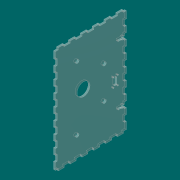
# Autodesk Inventor part: leftSide
Saved by Autodesk Inventor 2016 (Build 200138000, 138)
## iProperties
Created: 2015-10-05
Part Number: leftSide
Material: Polycarbonate, Clear
Document SubType Name: Modeling
Designer: Sawaiz
Density: 1.2 g/cm^3
Appearance: Polycarbonate - Clear
Author: Sawaiz
Autodesk Inventor part; units mm, degrees
ref_plane "YZ Plane" through (0, 0, 0) normal (1, 0, 0) x (0, 1, 0)
ref_plane "XZ Plane" through (0, 0, 0) normal (0, 1, 0) x (-1, 0, 0)
ref_plane "XY Plane" through (0, 0, 0) normal (0, 0, 1) x (1, 0, 0)
sketch "Sketch1" plane through (0, 0, 0) normal (1, 0, 0) x (0, 1, 0)
  line L0 (-56.825, -86.825) -> (56.825, -86.825)
  line L1 (56.825, -86.825) -> (56.825, 86.825)
  line L2 (56.825, 86.825) -> (-56.825, 86.825)
  line L3 (-56.825, 86.825) -> (-56.825, -86.825)
  line L4 (-56.825, -86.825) -> (56.825, 86.825) construction
  line L5 (56.825, -86.825) -> (-56.825, 86.825) construction
  point P0 (0, 0)
  dimension "d0" = 113.65
  dimension "d1" = 173.65
  constraints: 12 end point, 2 midpoint, 2 parallel, 1 horizontal, 1 perpendicular
  measures "d0" distance of L2.end L1.end
  measures "d1" distance of L1.end L0.end
extrude "Extrusion1" add sketch "Sketch1" along normal blind 3.175
sketch "Sketch10" plane through (0, 0, 0) normal (-1, 0, 0) x (0, 0, 1)
  line L0 (-86.825, -56.825) -> (-86.825, 56.825) projected
  line L1 (86.825, -56.825) -> (-86.825, -56.825) projected
  line L2 (86.825, 56.825) -> (86.825, -56.825) projected
  line L3 (-86.825, 56.825) -> (86.825, 56.825) projected
  line L4 (86.825, 56.825) -> (86.825, -56.825) projected
  line L5 (86.825, -55) -> (90, -55)
  line L6 (90, -55) -> (90, -45)
  line L7 (90, -45) -> (86.825, -45)
  line L8 (86.825, -45) -> (86.825, -55)
  point P0 (0, 0)
  dimension "d84" = 10
  dimension "d85" = 1.825
  dimension "d86" = 3.175
  constraints: 8 end point, 2 parallel, 1 horizontal, 1 perpendicular, 1 point on line
  measures "d84" distance of L5.end L6.end
  measures "d85" distance between parallel lines of L1 L5
  measures "d86" distance of L6.end L7.end
extrude "Extrusion4" add sketch "Sketch10" against normal up to surface (3.175 mm away) contours L2 L7 L6 L5
pattern_linear "Rectangular Pattern3" count 6 spacing 20 along (0, 1, 0) of "Extrusion4"
mirror "Mirror3" about plane through (0, 0, 0) normal (0, 0, 1) of "Extrusion4", "Rectangular Pattern3"
sketch "Sketch11" plane through (0, 0, 0) normal (-1, 0, 0) x (0, 0, 1)
  line L0 (-86.825, -56.825) -> (-86.825, -55) projected
  line L1 (86.825, -56.825) -> (-86.825, -56.825) projected
  line L2 (86.825, -55) -> (86.825, -56.825) projected
  line L3 (86.825, -55) -> (90, -55) projected
  line L4 (90, -55) -> (90, -45) projected
  line L5 (90, -45) -> (86.825, -45) projected
  line L6 (86.825, -35) -> (86.825, -45) projected
  line L7 (86.825, -35) -> (90, -35) projected
  line L8 (90, -35) -> (90, -25) projected
  line L9 (90, -25) -> (86.825, -25) projected
  line L10 (86.825, -15) -> (86.825, -25) projected
  line L11 (86.825, -15) -> (90, -15) projected
  line L12 (90, -15) -> (90, -5) projected
  line L13 (90, -5) -> (86.825, -5) projected
  line L14 (86.825, 5) -> (86.825, -5) projected
  line L15 (86.825, 5) -> (90, 5) projected
  line L16 (90, 5) -> (90, 15) projected
  line L17 (90, 15) -> (86.825, 15) projected
  line L18 (86.825, 25) -> (86.825, 15) projected
  line L19 (86.825, 25) -> (90, 25) projected
  line L20 (90, 25) -> (90, 35) projected
  line L21 (90, 35) -> (86.825, 35) projected
  line L22 (86.825, 45) -> (86.825, 35) projected
  line L23 (86.825, 45) -> (90, 45) projected
  line L24 (90, 45) -> (90, 55) projected
  line L25 (90, 55) -> (86.825, 55) projected
  line L26 (-86.825, 56.825) -> (86.825, 56.825) projected
  line L27 (-90, 55) -> (-86.825, 55) projected
  line L28 (-90, 45) -> (-90, 55) projected
  line L29 (-86.825, 45) -> (-90, 45) projected
  line L30 (-86.825, 35) -> (-86.825, 45) projected
  line L31 (-90, 35) -> (-86.825, 35) projected
  line L32 (-90, 25) -> (-90, 35) projected
  line L33 (-86.825, 25) -> (-90, 25) projected
  line L34 (-86.825, 15) -> (-86.825, 25) projected
  line L35 (-90, 15) -> (-86.825, 15) projected
  line L36 (-90, 5) -> (-90, 15) projected
  line L37 (-86.825, 5) -> (-90, 5) projected
  line L38 (-86.825, -5) -> (-86.825, 5) projected
  line L39 (-90, -5) -> (-86.825, -5) projected
  line L40 (-90, -15) -> (-90, -5) projected
  line L41 (-86.825, -15) -> (-90, -15) projected
  line L42 (-86.825, -25) -> (-86.825, -15) projected
  line L43 (-90, -25) -> (-86.825, -25) projected
  line L44 (-90, -35) -> (-90, -25) projected
  line L45 (-86.825, -35) -> (-90, -35) projected
  line L46 (-86.825, -45) -> (-86.825, -35) projected
  line L47 (-90, -45) -> (-86.825, -45) projected
  line L48 (-90, -55) -> (-90, -45) projected
  line L49 (-86.825, -55) -> (-90, -55) projected
  line L50 (86.825, -56.825) -> (-86.825, -56.825) projected
  line L51 (85, -56.825) -> (75, -56.825)
  line L52 (75, -56.825) -> (75, -60)
  line L53 (75, -60) -> (85, -60)
  line L54 (85, -60) -> (85, -56.825)
  line L55 (86.825, 56.825) -> (86.825, 55) projected
  line L56 (-86.825, 55) -> (-86.825, 56.825) projected
  point P0 (0, 0)
  dimension "d92" = 3.175
  dimension "d94" = 10
  dimension "d100" = 5
  constraints: 8 end point, 2 parallel, 1 horizontal, 1 perpendicular, 1 point on line
  measures "d92" distance of L53.end L51.start
  measures "d94" distance of L52.end L53.end
  measures "d100" distance between parallel lines of L4 L54
extrude "Extrusion5" add sketch "Sketch11" against normal up to surface (3.175 mm away) contours L1 L54 L53 L52
pattern_linear "Rectangular Pattern4" count 9 spacing 20 along (0, 0, -1) of "Extrusion5"
sketch "Sketch16" plane through (3.175, 0, 0) normal (1, 0, 0) x (0, 0, -1)
  line L0 (86.825, -56.825) -> (86.825, -55) projected
  line L1 (86.825, -55) -> (90, -55) projected
  line L2 (90, -55) -> (90, -45) projected
  line L3 (90, -45) -> (86.825, -45) projected
  line L4 (86.825, -45) -> (86.825, -35) projected
  line L5 (86.825, -35) -> (90, -35) projected
  line L6 (90, -35) -> (90, -25) projected
  line L7 (90, -25) -> (86.825, -25) projected
  line L8 (86.825, -25) -> (86.825, -15) projected
  line L9 (86.825, -15) -> (90, -15) projected
  line L10 (90, -15) -> (90, -5) projected
  line L11 (90, -5) -> (86.825, -5) projected
  line L12 (86.825, -5) -> (86.825, 5) projected
  line L13 (86.825, 5) -> (90, 5) projected
  line L14 (90, 5) -> (90, 15) projected
  line L15 (90, 15) -> (86.825, 15) projected
  line L16 (86.825, 15) -> (86.825, 25) projected
  line L17 (86.825, 25) -> (90, 25) projected
  line L18 (90, 25) -> (90, 35) projected
  line L19 (90, 35) -> (86.825, 35) projected
  line L20 (86.825, 35) -> (86.825, 45) projected
  line L21 (86.825, 45) -> (90, 45) projected
  line L22 (90, 45) -> (90, 55) projected
  line L23 (90, 55) -> (86.825, 55) projected
  line L24 (86.825, 55) -> (86.825, 56.825) projected
  line L25 (86.825, 56.825) -> (-86.825, 56.825) projected
  line L26 (-86.825, 56.825) -> (-86.825, 55) projected
  line L27 (-90, 55) -> (-86.825, 55) projected
  line L28 (-90, 45) -> (-90, 55) projected
  line L29 (-86.825, 45) -> (-90, 45) projected
  line L30 (-86.825, 45) -> (-86.825, 35) projected
  line L31 (-90, 35) -> (-86.825, 35) projected
  line L32 (-90, 25) -> (-90, 35) projected
  line L33 (-86.825, 25) -> (-90, 25) projected
  line L34 (-86.825, 25) -> (-86.825, 15) projected
  line L35 (-90, 15) -> (-86.825, 15) projected
  line L36 (-90, 5) -> (-90, 15) projected
  line L37 (-86.825, 5) -> (-90, 5) projected
  line L38 (-86.825, 5) -> (-86.825, -5) projected
  line L39 (-90, -5) -> (-86.825, -5) projected
  line L40 (-90, -15) -> (-90, -5) projected
  line L41 (-86.825, -15) -> (-90, -15) projected
  line L42 (-86.825, -15) -> (-86.825, -25) projected
  line L43 (-90, -25) -> (-86.825, -25) projected
  line L44 (-90, -35) -> (-90, -25) projected
  line L45 (-86.825, -35) -> (-90, -35) projected
  line L46 (-86.825, -35) -> (-86.825, -45) projected
  line L47 (-90, -45) -> (-86.825, -45) projected
  line L48 (-90, -55) -> (-90, -45) projected
  line L49 (-86.825, -55) -> (-90, -55) projected
  line L50 (-86.825, -55) -> (-86.825, -56.825) projected
  line L51 (-86.825, -56.825) -> (-85, -56.825) projected
  line L52 (-85, -60) -> (-85, -56.825) projected
  line L53 (-75, -60) -> (-85, -60) projected
  line L54 (-75, -56.825) -> (-75, -60) projected
  line L55 (-75, -56.825) -> (-65, -56.825) projected
  line L56 (-65, -60) -> (-65, -56.825) projected
  line L57 (-55, -60) -> (-65, -60) projected
  line L58 (-55, -56.825) -> (-55, -60) projected
  line L59 (-55, -56.825) -> (-45, -56.825) projected
  line L60 (-45, -60) -> (-45, -56.825) projected
  line L61 (-35, -60) -> (-45, -60) projected
  line L62 (-35, -56.825) -> (-35, -60) projected
  line L63 (-35, -56.825) -> (-25, -56.825) projected
  line L64 (-25, -60) -> (-25, -56.825) projected
  line L65 (-15, -60) -> (-25, -60) projected
  line L66 (-15, -56.825) -> (-15, -60) projected
  line L67 (-15, -56.825) -> (-5, -56.825) projected
  line L68 (-5, -60) -> (-5, -56.825) projected
  line L69 (5, -60) -> (-5, -60) projected
  line L70 (5, -56.825) -> (5, -60) projected
  line L71 (5, -56.825) -> (15, -56.825) projected
  line L72 (15, -60) -> (15, -56.825) projected
  line L73 (25, -60) -> (15, -60) projected
  line L74 (25, -56.825) -> (25, -60) projected
  line L75 (25, -56.825) -> (35, -56.825) projected
  line L76 (35, -60) -> (35, -56.825) projected
  line L77 (45, -60) -> (35, -60) projected
  line L78 (45, -56.825) -> (45, -60) projected
  line L79 (45, -56.825) -> (55, -56.825) projected
  line L80 (55, -60) -> (55, -56.825) projected
  line L81 (65, -60) -> (55, -60) projected
  line L82 (65, -56.825) -> (65, -60) projected
  line L83 (65, -56.825) -> (75, -56.825) projected
  line L84 (75, -60) -> (75, -56.825) projected
  line L85 (85, -60) -> (75, -60) projected
  line L86 (85, -56.825) -> (85, -60) projected
  line L87 (85, -56.825) -> (86.825, -56.825) projected
  line L88 (-85, -56.825) -> (-86.825, -56.825)
  line L89 (-86.825, -56.825) -> (-86.825, -60)
  line L90 (-86.825, -60) -> (-85, -60)
  line L91 (-85, -60) -> (-85, -56.825)
  line L92 (85, -56.825) -> (85, -60) projected
  line L93 (85, -56.825) -> (86.825, -56.825)
  line L94 (86.825, -56.825) -> (86.825, -60)
  line L95 (86.825, -60) -> (85, -60)
  line L96 (85, -60) -> (85, -56.825)
  point P0 (0, 0)
  constraints: 16 end point, 4 collinear, 4 parallel, 2 horizontal, 2 perpendicular
extrude "Extrusion8" add sketch "Sketch16" against normal up to surface (3.175 mm away) contours L94 L95 L86 L87 | L90 L89 L51 L52
mirror "Mirror4" about plane through (0, 0, 0) normal (0, 1, 0) of "Extrusion5", "Rectangular Pattern4", "Extrusion8"
sketch "Sketch2" plane through (3.175, 0, 0) normal (1, 0, 0) x (0, 0, -1)
  line L0 (86.825, -60) -> (86.825, -55) projected
  line L1 (-65, 56.825) -> (-75, 56.825) projected
  line L2 (-86.825, 55) -> (-86.825, 60) projected
  line L3 (-75, -56.825) -> (-65, -56.825) projected
  line L4 (-86.825, 56.825) -> (-86.825, -56.825) projected
  line L5 (86.825, -55) -> (90, -55) projected
  line L6 (90, -55) -> (90, -45) projected
  line L7 (90, -45) -> (86.825, -45) projected
  line L8 (86.825, -45) -> (86.825, -35) projected
  line L9 (86.825, -35) -> (90, -35) projected
  line L10 (90, -35) -> (90, -25) projected
  line L11 (90, -25) -> (86.825, -25) projected
  line L12 (86.825, -15) -> (90, -15) projected
  line L13 (90, -15) -> (90, -5) projected
  line L14 (90, -5) -> (86.825, -5) projected
  line L15 (86.825, -5) -> (86.825, 5) projected
  line L16 (86.825, 5) -> (90, 5) projected
  line L17 (90, 5) -> (90, 15) projected
  line L18 (90, 15) -> (86.825, 15) projected
  line L19 (86.825, 15) -> (86.825, 25) projected
  line L20 (86.825, 25) -> (90, 25) projected
  line L21 (90, 25) -> (90, 35) projected
  line L22 (90, 35) -> (86.825, 35) projected
  line L23 (86.825, 35) -> (86.825, 45) projected
  line L24 (86.825, 45) -> (90, 45) projected
  line L25 (90, 45) -> (90, 55) projected
  line L26 (90, 55) -> (86.825, 55) projected
  line L27 (86.825, 60) -> (75, 60) projected
  line L28 (75, 60) -> (75, 56.825) projected
  line L29 (65, 56.825) -> (65, 60) projected
  line L30 (65, 60) -> (55, 60) projected
  line L31 (55, 60) -> (55, 56.825) projected
  line L32 (55, 56.825) -> (45, 56.825) projected
  line L33 (45, 56.825) -> (45, 60) projected
  line L34 (45, 60) -> (35, 60) projected
  line L35 (35, 60) -> (35, 56.825) projected
  line L36 (35, 56.825) -> (25, 56.825) projected
  line L37 (25, 56.825) -> (25, 60) projected
  line L38 (25, 60) -> (15, 60) projected
  line L39 (15, 60) -> (15, 56.825) projected
  line L40 (15, 56.825) -> (5, 56.825) projected
  line L41 (5, 56.825) -> (5, 60) projected
  line L42 (5, 60) -> (-5, 60) projected
  line L43 (-5, 60) -> (-5, 56.825) projected
  line L44 (-5, 56.825) -> (-15, 56.825) projected
  line L45 (-15, 56.825) -> (-15, 60) projected
  line L46 (-15, 60) -> (-25, 60) projected
  line L47 (-25, 60) -> (-25, 56.825) projected
  line L48 (-25, 56.825) -> (-35, 56.825) projected
  line L49 (-35, 56.825) -> (-35, 60) projected
  line L50 (-35, 60) -> (-45, 60) projected
  line L51 (-45, 60) -> (-45, 56.825) projected
  line L52 (-45, 56.825) -> (-55, 56.825) projected
  line L53 (-55, 56.825) -> (-55, 60) projected
  line L54 (-55, 60) -> (-65, 60) projected
  line L55 (-65, 60) -> (-65, 56.825) projected
  line L56 (-75, 56.825) -> (-75, 60) projected
  line L57 (-75, 60) -> (-86.825, 60) projected
  line L58 (-90, 55) -> (-86.825, 55) projected
  line L59 (-90, 45) -> (-90, 55) projected
  line L60 (-86.825, 45) -> (-90, 45) projected
  line L61 (-86.825, 45) -> (-86.825, 35) projected
  line L62 (-90, 35) -> (-86.825, 35) projected
  line L63 (-90, 25) -> (-90, 35) projected
  line L64 (-86.825, 25) -> (-90, 25) projected
  line L65 (-86.825, 25) -> (-86.825, 15) projected
  line L66 (-90, 15) -> (-86.825, 15) projected
  line L67 (-90, 5) -> (-90, 15) projected
  line L68 (-86.825, 5) -> (-90, 5) projected
  line L69 (-86.825, 5) -> (-86.825, -5) projected
  line L70 (-90, -5) -> (-86.825, -5) projected
  line L71 (-90, -15) -> (-90, -5) projected
  line L72 (-86.825, -15) -> (-90, -15) projected
  line L73 (-86.825, -15) -> (-86.825, -25) projected
  line L74 (-90, -25) -> (-86.825, -25) projected
  line L75 (-90, -35) -> (-90, -25) projected
  line L76 (-86.825, -35) -> (-90, -35) projected
  line L77 (-86.825, -35) -> (-86.825, -45) projected
  line L78 (-90, -45) -> (-86.825, -45) projected
  line L79 (-90, -55) -> (-90, -45) projected
  line L80 (-86.825, -55) -> (-90, -55) projected
  line L81 (-75, -60) -> (-86.825, -60) projected
  line L82 (-75, -56.825) -> (-75, -60) projected
  line L83 (-65, -60) -> (-65, -56.825) projected
  line L84 (-55, -60) -> (-65, -60) projected
  line L85 (-55, -56.825) -> (-55, -60) projected
  line L86 (-55, -56.825) -> (-45, -56.825) projected
  line L87 (-45, -60) -> (-45, -56.825) projected
  line L88 (-35, -60) -> (-45, -60) projected
  line L89 (-35, -56.825) -> (-35, -60) projected
  line L90 (-35, -56.825) -> (-25, -56.825) projected
  line L91 (-25, -60) -> (-25, -56.825) projected
  line L92 (-15, -60) -> (-25, -60) projected
  line L93 (-15, -56.825) -> (-15, -60) projected
  line L94 (-15, -56.825) -> (-5, -56.825) projected
  line L95 (-5, -60) -> (-5, -56.825) projected
  line L96 (5, -60) -> (-5, -60) projected
  line L97 (5, -56.825) -> (5, -60) projected
  line L98 (5, -56.825) -> (15, -56.825) projected
  line L99 (15, -60) -> (15, -56.825) projected
  line L100 (25, -60) -> (15, -60) projected
  line L101 (25, -56.825) -> (25, -60) projected
  line L102 (25, -56.825) -> (35, -56.825) projected
  line L103 (35, -60) -> (35, -56.825) projected
  line L104 (45, -60) -> (35, -60) projected
  line L105 (45, -56.825) -> (45, -60) projected
  line L106 (45, -56.825) -> (55, -56.825) projected
  line L107 (55, -60) -> (55, -56.825) projected
  line L108 (65, -60) -> (55, -60) projected
  line L109 (65, -56.825) -> (65, -60) projected
  line L110 (65, -56.825) -> (75, -56.825) projected
  line L111 (75, -60) -> (75, -56.825) projected
  line L112 (75, -60) -> (86.825, -60) projected
  line L113 (75, 56.825) -> (65, 56.825) projected
  line L114 (86.825, 55) -> (86.825, 60) projected
  line L115 (-86.825, -55) -> (-86.825, -60) projected
  line L116 (86.825, -25) -> (86.825, -15) projected
  point P0 (0, 0)
  point P1 (-8.175, -15)
  dimension "d4" = 95
  dimension "d12" = 41.825
  measures "d4" distance from line of L0 point (-8.175, -15)
  measures "d12" distance from line of L3 point (-8.175, -15)
hole "Hole1" at (3.175, -15, 8.175) direction (-1, 0, 0) diameter 22 end through all
sketch "Sketch6" plane through (3.175, 0, 0) normal (1, 0, 0) x (0, 0, -1)
  circle A0 centre (-8.175, -15) radius 11 projected
  line L0 (86.825, -60) -> (86.825, -55) projected
  line L1 (-65, 56.825) -> (-75, 56.825) projected
  line L2 (-86.825, 55) -> (-86.825, 60) projected
  line L3 (-75, -56.825) -> (-65, -56.825) projected
  line L4 (-86.825, -56.825) -> (86.825, -56.825) projected
  line L5 (-48.5, 56.825) -> (-48.5, 54.825)
  line L6 (-48.5, 54.825) -> (-47.25, 54.825)
  line L7 (-47.25, 54.825) -> (-47.25, 52.325)
  line L8 (-47.25, 52.325) -> (-48.5, 52.325)
  line L9 (-48.5, 52.325) -> (-48.5, 46)
  line L10 (-48.5, 46) -> (-51.5, 46)
  line L11 (-51.5, 46) -> (-51.5, 52.325)
  line L12 (-51.5, 52.325) -> (-52.75, 52.325)
  line L13 (-52.75, 52.325) -> (-52.75, 54.825)
  line L14 (-52.75, 54.825) -> (-51.5, 54.825)
  line L15 (-51.5, 56.825) -> (-51.5, 54.825)
  line L16 (86.825, -55) -> (90, -55) projected
  line L17 (90, -55) -> (90, -45) projected
  line L18 (90, -45) -> (86.825, -45) projected
  line L19 (86.825, -45) -> (86.825, -35) projected
  line L20 (86.825, -35) -> (90, -35) projected
  line L21 (90, -35) -> (90, -25) projected
  line L22 (90, -25) -> (86.825, -25) projected
  line L23 (86.825, -15) -> (90, -15) projected
  line L24 (90, -15) -> (90, -5) projected
  line L25 (90, -5) -> (86.825, -5) projected
  line L26 (86.825, -5) -> (86.825, 5) projected
  line L27 (86.825, 5) -> (90, 5) projected
  line L28 (90, 5) -> (90, 15) projected
  line L29 (90, 15) -> (86.825, 15) projected
  line L30 (86.825, 15) -> (86.825, 25) projected
  line L31 (86.825, 25) -> (90, 25) projected
  line L32 (90, 25) -> (90, 35) projected
  line L33 (90, 35) -> (86.825, 35) projected
  line L34 (86.825, 35) -> (86.825, 45) projected
  line L35 (86.825, 45) -> (90, 45) projected
  line L36 (90, 45) -> (90, 55) projected
  line L37 (90, 55) -> (86.825, 55) projected
  line L38 (86.825, 60) -> (75, 60) projected
  line L39 (75, 60) -> (75, 56.825) projected
  line L40 (75, 56.825) -> (65, 56.825) projected
  line L41 (65, 56.825) -> (65, 60) projected
  line L42 (65, 60) -> (55, 60) projected
  line L43 (55, 60) -> (55, 56.825) projected
  line L44 (55, 56.825) -> (45, 56.825) projected
  line L45 (45, 56.825) -> (45, 60) projected
  line L46 (45, 60) -> (35, 60) projected
  line L47 (35, 60) -> (35, 56.825) projected
  line L48 (25, 56.825) -> (25, 60) projected
  line L49 (25, 60) -> (15, 60) projected
  line L50 (15, 60) -> (15, 56.825) projected
  line L51 (15, 56.825) -> (5, 56.825) projected
  line L52 (5, 56.825) -> (5, 60) projected
  line L53 (5, 60) -> (-5, 60) projected
  line L54 (-5, 60) -> (-5, 56.825) projected
  line L55 (-5, 56.825) -> (-15, 56.825) projected
  line L56 (-15, 56.825) -> (-15, 60) projected
  line L57 (-15, 60) -> (-25, 60) projected
  line L58 (-25, 60) -> (-25, 56.825) projected
  line L59 (-25, 56.825) -> (-35, 56.825) projected
  line L60 (-35, 56.825) -> (-35, 60) projected
  line L61 (-35, 60) -> (-45, 60) projected
  line L62 (-45, 60) -> (-45, 56.825) projected
  line L63 (-45, 56.825) -> (-55, 56.825) projected
  line L64 (-55, 56.825) -> (-55, 60) projected
  line L65 (-55, 60) -> (-65, 60) projected
  line L66 (-65, 60) -> (-65, 56.825) projected
  line L67 (-75, 56.825) -> (-75, 60) projected
  line L68 (-75, 60) -> (-86.825, 60) projected
  line L69 (-90, 55) -> (-86.825, 55) projected
  line L70 (-90, 45) -> (-90, 55) projected
  line L71 (-86.825, 45) -> (-90, 45) projected
  line L72 (-86.825, 45) -> (-86.825, 35) projected
  line L73 (-90, 35) -> (-86.825, 35) projected
  line L74 (-90, 25) -> (-90, 35) projected
  line L75 (-86.825, 25) -> (-90, 25) projected
  line L76 (-90, 15) -> (-86.825, 15) projected
  line L77 (-90, 5) -> (-90, 15) projected
  line L78 (-86.825, 5) -> (-90, 5) projected
  line L79 (-86.825, 5) -> (-86.825, -5) projected
  line L80 (-90, -5) -> (-86.825, -5) projected
  line L81 (-90, -15) -> (-90, -5) projected
  line L82 (-86.825, -15) -> (-90, -15) projected
  line L83 (-86.825, -15) -> (-86.825, -25) projected
  line L84 (-90, -25) -> (-86.825, -25) projected
  line L85 (-90, -35) -> (-90, -25) projected
  line L86 (-86.825, -35) -> (-90, -35) projected
  line L87 (-86.825, -35) -> (-86.825, -45) projected
  line L88 (-90, -45) -> (-86.825, -45) projected
  line L89 (-90, -55) -> (-90, -45) projected
  line L90 (-86.825, -55) -> (-90, -55) projected
  line L91 (-75, -60) -> (-86.825, -60) projected
  line L92 (-75, -56.825) -> (-75, -60) projected
  line L93 (-65, -60) -> (-65, -56.825) projected
  line L94 (-55, -60) -> (-65, -60) projected
  line L95 (-55, -56.825) -> (-55, -60) projected
  line L96 (-55, -56.825) -> (-45, -56.825) projected
  line L97 (-45, -60) -> (-45, -56.825) projected
  line L98 (-35, -60) -> (-45, -60) projected
  line L99 (-35, -56.825) -> (-35, -60) projected
  line L100 (-35, -56.825) -> (-25, -56.825) projected
  line L101 (-25, -60) -> (-25, -56.825) projected
  line L102 (-15, -60) -> (-25, -60) projected
  line L103 (-15, -56.825) -> (-15, -60) projected
  line L104 (-5, -60) -> (-5, -56.825) projected
  line L105 (5, -60) -> (-5, -60) projected
  line L106 (5, -56.825) -> (5, -60) projected
  line L107 (5, -56.825) -> (15, -56.825) projected
  line L108 (15, -60) -> (15, -56.825) projected
  line L109 (25, -60) -> (15, -60) projected
  line L110 (25, -56.825) -> (25, -60) projected
  line L111 (25, -56.825) -> (35, -56.825) projected
  line L112 (35, -60) -> (35, -56.825) projected
  line L113 (45, -60) -> (35, -60) projected
  line L114 (45, -56.825) -> (45, -60) projected
  line L115 (45, -56.825) -> (55, -56.825) projected
  line L116 (55, -60) -> (55, -56.825) projected
  line L117 (65, -60) -> (55, -60) projected
  line L118 (65, -56.825) -> (65, -60) projected
  line L119 (65, -56.825) -> (75, -56.825) projected
  line L120 (75, -60) -> (75, -56.825) projected
  line L121 (75, -60) -> (86.825, -60) projected
  line L122 (-86.825, 25) -> (-86.825, 15) projected
  line L123 (-15, -56.825) -> (-5, -56.825) projected
  line L124 (-51.5, 56.825) -> (-48.5, 56.825)
  line L125 (35, 56.825) -> (25, 56.825) projected
  line L126 (86.825, 55) -> (86.825, 60) projected
  line L127 (-86.825, -55) -> (-86.825, -60) projected
  line L128 (86.825, -25) -> (86.825, -15) projected
  point P0 (0, 0)
  point P1 (-50, 46)
  dimension "d40" = 3
  dimension "d41" = 5.5
  dimension "d42" = 2.5
  dimension "d101" = 10.825
  dimension "d103" = 2
  dimension "d104" = 2
  dimension "d105" = 50
  constraints: 24 end point, 8 point on line, 6 perpendicular, 1 collinear, 1 midpoint, 1 vertical
  measures "d40" distance between parallel lines of L15 L5
  measures "d41" distance between parallel lines of L7 L13
  measures "d42" distance between parallel lines of L14 L12
  measures "d101" distance from line of L5.start L10
  measures "d103" distance from line of L14 L15.start
  measures "d104" distance from line of L5.start L6
  measures "d105" horizontal distance of point (0, 0) point (-50, 46)
sketch "Sketch9" plane through (3.175, 0, 0) normal (1, 0, 0) x (0, 0, -1)
  line L0 (54, -22.9972) -> (-54, -22.9972)
  line L1 (-54, -22.9972) -> (-27.4451, 22.9972)
  line L2 (-27.4451, 22.9972) -> (27.4451, 22.9972)
  line L3 (27.4451, 22.9972) -> (54, -22.9972)
  line L4 (-45, -60) -> (-45, -56.825) projected
  line L5 (-35, -60) -> (-45, -60) projected
  line L6 (-35, -56.825) -> (-35, -60) projected
  line L7 (-25, -60) -> (-25, -56.825) projected
  line L8 (-15, -60) -> (-25, -60) projected
  line L9 (-15, -56.825) -> (-15, -60) projected
  line L10 (-5, -60) -> (-5, -56.825) projected
  line L11 (5, -60) -> (-5, -60) projected
  line L12 (5, -56.825) -> (5, -60) projected
  line L13 (15, -60) -> (15, -56.825) projected
  line L14 (25, -60) -> (15, -60) projected
  line L15 (25, -56.825) -> (25, -60) projected
  line L16 (35, -60) -> (35, -56.825) projected
  line L17 (45, -60) -> (35, -60) projected
  line L18 (45, -56.825) -> (45, -60) projected
  line L19 (55, -60) -> (55, -56.825) projected
  line L20 (65, -60) -> (55, -60) projected
  line L21 (65, -56.825) -> (65, -60) projected
  line L22 (75, -60) -> (75, -56.825) projected
  line L23 (75, -60) -> (86.825, -60) projected
  line L24 (-75, -60) -> (-86.825, -60) projected
  line L25 (-75, -56.825) -> (-75, -60) projected
  line L26 (-65, -60) -> (-65, -56.825) projected
  line L27 (-55, -60) -> (-65, -60) projected
  line L28 (-55, -56.825) -> (-55, -60) projected
  line L29 (86.825, -25) -> (86.825, -15) projected
  line L30 (86.825, -55) -> (90, -55) projected
  line L31 (90, -55) -> (90, -45) projected
  line L32 (90, -45) -> (86.825, -45) projected
  line L33 (86.825, -45) -> (86.825, -35) projected
  line L34 (86.825, -35) -> (90, -35) projected
  line L35 (90, -35) -> (90, -25) projected
  line L36 (90, -25) -> (86.825, -25) projected
  line L37 (86.825, -15) -> (90, -15) projected
  line L38 (90, -15) -> (90, -5) projected
  line L39 (90, -5) -> (86.825, -5) projected
  line L40 (86.825, -5) -> (86.825, 5) projected
  line L41 (86.825, 5) -> (90, 5) projected
  line L42 (90, 5) -> (90, 15) projected
  line L43 (90, 15) -> (86.825, 15) projected
  line L44 (86.825, 15) -> (86.825, 25) projected
  line L45 (86.825, 25) -> (90, 25) projected
  line L46 (90, 25) -> (90, 35) projected
  line L47 (90, 35) -> (86.825, 35) projected
  line L48 (86.825, 35) -> (86.825, 45) projected
  line L49 (86.825, 45) -> (90, 45) projected
  line L50 (90, 45) -> (90, 55) projected
  line L51 (90, 55) -> (86.825, 55) projected
  line L52 (-65, 56.825) -> (-75, 56.825) projected
  line L53 (86.825, 60) -> (75, 60) projected
  line L54 (75, 60) -> (75, 56.825) projected
  line L55 (65, 56.825) -> (65, 60) projected
  line L56 (65, 60) -> (55, 60) projected
  line L57 (55, 60) -> (55, 56.825) projected
  line L58 (55, 56.825) -> (45, 56.825) projected
  line L59 (45, 56.825) -> (45, 60) projected
  line L60 (45, 60) -> (35, 60) projected
  line L61 (35, 60) -> (35, 56.825) projected
  line L62 (35, 56.825) -> (25, 56.825) projected
  line L63 (25, 56.825) -> (25, 60) projected
  line L64 (25, 60) -> (15, 60) projected
  line L65 (15, 60) -> (15, 56.825) projected
  line L66 (15, 56.825) -> (5, 56.825) projected
  line L67 (5, 56.825) -> (5, 60) projected
  line L68 (5, 60) -> (-5, 60) projected
  line L69 (-5, 60) -> (-5, 56.825) projected
  line L70 (-5, 56.825) -> (-15, 56.825) projected
  line L71 (-15, 56.825) -> (-15, 60) projected
  line L72 (-15, 60) -> (-25, 60) projected
  line L73 (-25, 60) -> (-25, 56.825) projected
  line L74 (-25, 56.825) -> (-35, 56.825) projected
  line L75 (-35, 56.825) -> (-35, 60) projected
  line L76 (-35, 60) -> (-45, 60) projected
  line L77 (-45, 60) -> (-45, 56.825) projected
  line L78 (-45, 56.825) -> (-55, 56.825) projected
  line L79 (-55, 56.825) -> (-55, 60) projected
  line L80 (-55, 60) -> (-65, 60) projected
  line L81 (-65, 60) -> (-65, 56.825) projected
  line L82 (-75, 56.825) -> (-75, 60) projected
  line L83 (-75, 60) -> (-86.825, 60) projected
  line L84 (-86.825, -35) -> (-86.825, -45) projected
  line L85 (-90, 55) -> (-86.825, 55) projected
  line L86 (-90, 45) -> (-90, 55) projected
  line L87 (-86.825, 45) -> (-90, 45) projected
  line L88 (-86.825, 45) -> (-86.825, 35) projected
  line L89 (-90, 35) -> (-86.825, 35) projected
  line L90 (-90, 25) -> (-90, 35) projected
  line L91 (-86.825, 25) -> (-90, 25) projected
  line L92 (-86.825, 25) -> (-86.825, 15) projected
  line L93 (-90, 15) -> (-86.825, 15) projected
  line L94 (-90, 5) -> (-90, 15) projected
  line L95 (-86.825, 5) -> (-90, 5) projected
  line L96 (-86.825, 5) -> (-86.825, -5) projected
  line L97 (-90, -5) -> (-86.825, -5) projected
  line L98 (-90, -15) -> (-90, -5) projected
  line L99 (-86.825, -15) -> (-90, -15) projected
  line L100 (-90, -25) -> (-86.825, -25) projected
  line L101 (-90, -35) -> (-90, -25) projected
  line L102 (-86.825, -35) -> (-90, -35) projected
  line L103 (-90, -45) -> (-86.825, -45) projected
  line L104 (-90, -55) -> (-90, -45) projected
  line L105 (-86.825, -55) -> (-90, -55) projected
  line L106 (-75, -56.825) -> (-65, -56.825) projected
  line L107 (-55, -56.825) -> (-45, -56.825) projected
  line L108 (-35, -56.825) -> (-25, -56.825) projected
  line L109 (-15, -56.825) -> (-5, -56.825) projected
  line L110 (5, -56.825) -> (15, -56.825) projected
  line L111 (25, -56.825) -> (35, -56.825) projected
  line L112 (45, -56.825) -> (55, -56.825) projected
  line L113 (65, -56.825) -> (75, -56.825) projected
  line L114 (-86.825, -15) -> (-86.825, -25) projected
  line L115 (86.825, -60) -> (86.825, -55) projected
  line L116 (86.825, 55) -> (86.825, 60) projected
  line L117 (-86.825, 55) -> (-86.825, 60) projected
  line L118 (-86.825, -55) -> (-86.825, -60) projected
  line L119 (75, 56.825) -> (65, 56.825) projected
  point P0 (0, 0)
  dimension "d74" = 60
  dimension "d75" = 60
  constraints: 8 end point, 2 horizontal
  measures "d74" angle of L0 L1
  measures "d75" angle of L0 L3
hole "Hole6" at (3.175, -22.9972, 54) at (3.175, 22.9972, 27.4451) at (3.175, 22.9972, -27.4451) at (3.175, -22.9972, -54) direction (-1, 0, 0) diameter 6 end through all
extrude "Extrusion6" cut sketch "Sketch6" against normal through all contours L63 L5 L6 L7 L8 L9 L10 L11 L12 L13 L14 L15
mirror "Mirror5" about plane through (0, 0, 0) normal (0, 0, 1) of "Extrusion6"
sketch "Sketch14" plane through (0, 0, 0) normal (-1, 0, 0) x (0, 0, 1)
  line L0 (-15.24, 45.72) -> (0, 45.72) construction
  line L1 (0, 45.72) -> (0, 0) construction
  line L2 (-15.24, 38.1) -> (-15.24, 45.72) construction
  line L3 (-15.24, 38.1) -> (0, 38.1) construction
  dimension "d127" = 45.72
  dimension "d128" = 15.24
  dimension "d142" = 7.62
  constraints: 8 end point, 2 horizontal, 1 perpendicular, 1 point on line, 1 vertical
  measures "d127" distance of L0.end L1.end
  measures "d128" distance of L0.start L0.end
  measures "d142" distance of L2.start L0.start
hole "Hole9" at (0, 45.72, 0) at (0, 45.72, -15.24) at (0, 38.1, -15.24) at (0, 38.1, 0) direction (1, 0, 0) diameter 2.156 end through all thread size "4-40 UNC" class "2B" standard "ANSI Unified Screw Threads"
sketch "Sketch15" plane through (0, 0, 0) normal (-1, 0, 0) x (0, 0, 1)
  line L0 (-1.905, 43.815) -> (-13.335, 43.815)
  line L1 (-13.335, 43.815) -> (-13.335, 40.005)
  line L2 (-13.335, 40.005) -> (-1.905, 40.005)
  line L3 (-1.905, 40.005) -> (-1.905, 43.815)
  circle A0 centre (0, 45.72) radius 1.078 projected
  circle A1 centre (-15.24, 45.72) radius 1.078 projected
  circle A2 centre (-27.4451, 22.9972) radius 3 projected
  circle A3 centre (54, -22.9972) radius 3 projected
  circle A4 centre (27.4451, 22.9972) radius 3 projected
  circle A5 centre (-54, -22.9972) radius 3 projected
  circle A6 centre (8.175, -15) radius 11 projected
  line L4 (-48.5, 56.825) -> (-48.5, 54.825) projected
  line L5 (-48.5, 54.825) -> (-47.25, 54.825) projected
  line L6 (-47.25, 54.825) -> (-47.25, 52.325) projected
  line L7 (-47.25, 52.325) -> (-48.5, 52.325) projected
  line L8 (-48.5, 52.325) -> (-48.5, 46) projected
  line L9 (-48.5, 46) -> (-51.5, 46) projected
  line L10 (-51.5, 46) -> (-51.5, 52.325) projected
  line L11 (-51.5, 52.325) -> (-52.75, 52.325) projected
  line L12 (-52.75, 52.325) -> (-52.75, 54.825) projected
  line L13 (-52.75, 54.825) -> (-51.5, 54.825) projected
  line L14 (-51.5, 54.825) -> (-51.5, 56.825) projected
  line L15 (-55, 56.825) -> (-51.5, 56.825) projected
  line L16 (-55, 60) -> (-55, 56.825) projected
  line L17 (-65, 60) -> (-55, 60) projected
  line L18 (-65, 56.825) -> (-65, 60) projected
  line L19 (-75, 56.825) -> (-65, 56.825) projected
  line L20 (-75, 60) -> (-75, 56.825) projected
  line L21 (65, 56.825) -> (75, 56.825) projected
  line L22 (-86.825, -45) -> (-86.825, -35) projected
  line L23 (-90, 55) -> (-86.825, 55) projected
  line L24 (-90, 45) -> (-90, 55) projected
  line L25 (-86.825, 45) -> (-90, 45) projected
  line L26 (-86.825, 35) -> (-86.825, 45) projected
  line L27 (-90, 35) -> (-86.825, 35) projected
  line L28 (-90, 25) -> (-90, 35) projected
  line L29 (-86.825, 25) -> (-90, 25) projected
  line L30 (-86.825, 15) -> (-86.825, 25) projected
  line L31 (-90, 15) -> (-86.825, 15) projected
  line L32 (-90, 5) -> (-90, 15) projected
  line L33 (-86.825, 5) -> (-90, 5) projected
  line L34 (-86.825, -5) -> (-86.825, 5) projected
  line L35 (-90, -5) -> (-86.825, -5) projected
  line L36 (-90, -15) -> (-90, -5) projected
  line L37 (-86.825, -15) -> (-90, -15) projected
  line L38 (-86.825, -25) -> (-86.825, -15) projected
  line L39 (-90, -25) -> (-86.825, -25) projected
  line L40 (-90, -35) -> (-90, -25) projected
  line L41 (-86.825, -35) -> (-90, -35) projected
  line L42 (-90, -45) -> (-86.825, -45) projected
  line L43 (-90, -55) -> (-90, -45) projected
  line L44 (-86.825, -55) -> (-90, -55) projected
  line L45 (75, -56.825) -> (65, -56.825) projected
  line L46 (-75, -60) -> (-75, -56.825) projected
  line L47 (-65, -56.825) -> (-75, -56.825) projected
  line L48 (-65, -56.825) -> (-65, -60) projected
  line L49 (-65, -60) -> (-55, -60) projected
  line L50 (-55, -60) -> (-55, -56.825) projected
  line L51 (-45, -56.825) -> (-55, -56.825) projected
  line L52 (-45, -56.825) -> (-45, -60) projected
  line L53 (-45, -60) -> (-35, -60) projected
  line L54 (-35, -60) -> (-35, -56.825) projected
  line L55 (-25, -56.825) -> (-35, -56.825) projected
  line L56 (-25, -56.825) -> (-25, -60) projected
  line L57 (-25, -60) -> (-15, -60) projected
  line L58 (-15, -60) -> (-15, -56.825) projected
  line L59 (-5, -56.825) -> (-15, -56.825) projected
  line L60 (-5, -56.825) -> (-5, -60) projected
  line L61 (-5, -60) -> (5, -60) projected
  line L62 (5, -60) -> (5, -56.825) projected
  line L63 (15, -56.825) -> (5, -56.825) projected
  line L64 (15, -56.825) -> (15, -60) projected
  line L65 (15, -60) -> (25, -60) projected
  line L66 (25, -60) -> (25, -56.825) projected
  line L67 (35, -56.825) -> (25, -56.825) projected
  line L68 (35, -56.825) -> (35, -60) projected
  line L69 (35, -60) -> (45, -60) projected
  line L70 (45, -60) -> (45, -56.825) projected
  line L71 (55, -56.825) -> (45, -56.825) projected
  line L72 (55, -56.825) -> (55, -60) projected
  line L73 (55, -60) -> (65, -60) projected
  line L74 (65, -60) -> (65, -56.825) projected
  line L75 (75, -56.825) -> (75, -60) projected
  line L76 (86.825, -35) -> (86.825, -45) projected
  line L77 (86.825, -55) -> (90, -55) projected
  line L78 (90, -55) -> (90, -45) projected
  line L79 (90, -45) -> (86.825, -45) projected
  line L80 (86.825, -35) -> (90, -35) projected
  line L81 (90, -35) -> (90, -25) projected
  line L82 (90, -25) -> (86.825, -25) projected
  line L83 (86.825, -15) -> (86.825, -25) projected
  line L84 (86.825, -15) -> (90, -15) projected
  line L85 (90, -15) -> (90, -5) projected
  line L86 (90, -5) -> (86.825, -5) projected
  line L87 (86.825, 5) -> (86.825, -5) projected
  line L88 (86.825, 5) -> (90, 5) projected
  line L89 (90, 5) -> (90, 15) projected
  line L90 (90, 15) -> (86.825, 15) projected
  line L91 (86.825, 25) -> (86.825, 15) projected
  line L92 (86.825, 25) -> (90, 25) projected
  line L93 (90, 25) -> (90, 35) projected
  line L94 (90, 35) -> (86.825, 35) projected
  line L95 (86.825, 45) -> (86.825, 35) projected
  line L96 (86.825, 45) -> (90, 45) projected
  line L97 (90, 45) -> (90, 55) projected
  line L98 (90, 55) -> (86.825, 55) projected
  line L99 (75, 56.825) -> (75, 60) projected
  line L100 (65, 60) -> (65, 56.825) projected
  line L101 (55, 60) -> (65, 60) projected
  line L102 (55, 56.825) -> (55, 60) projected
  line L103 (51.5, 56.825) -> (55, 56.825) projected
  line L104 (51.5, 56.825) -> (51.5, 54.825) projected
  line L105 (51.5, 54.825) -> (52.75, 54.825) projected
  line L106 (52.75, 54.825) -> (52.75, 52.325) projected
  line L107 (52.75, 52.325) -> (51.5, 52.325) projected
  line L108 (51.5, 52.325) -> (51.5, 46) projected
  line L109 (51.5, 46) -> (48.5, 46) projected
  line L110 (48.5, 46) -> (48.5, 52.325) projected
  line L111 (48.5, 52.325) -> (47.25, 52.325) projected
  line L112 (47.25, 52.325) -> (47.25, 54.825) projected
  line L113 (47.25, 54.825) -> (48.5, 54.825) projected
  line L114 (48.5, 54.825) -> (48.5, 56.825) projected
  line L115 (45, 56.825) -> (48.5, 56.825) projected
  line L116 (45, 60) -> (45, 56.825) projected
  line L117 (35, 60) -> (45, 60) projected
  line L118 (35, 56.825) -> (35, 60) projected
  line L119 (25, 56.825) -> (35, 56.825) projected
  line L120 (25, 60) -> (25, 56.825) projected
  line L121 (15, 60) -> (25, 60) projected
  line L122 (15, 56.825) -> (15, 60) projected
  line L123 (5, 56.825) -> (15, 56.825) projected
  line L124 (5, 60) -> (5, 56.825) projected
  line L125 (-5, 60) -> (5, 60) projected
  line L126 (-5, 56.825) -> (-5, 60) projected
  line L127 (-15, 56.825) -> (-5, 56.825) projected
  line L128 (-15, 60) -> (-15, 56.825) projected
  line L129 (-25, 60) -> (-15, 60) projected
  line L130 (-25, 56.825) -> (-25, 60) projected
  line L131 (-35, 56.825) -> (-25, 56.825) projected
  line L132 (-35, 60) -> (-35, 56.825) projected
  line L133 (-45, 60) -> (-35, 60) projected
  line L134 (-45, 56.825) -> (-45, 60) projected
  line L135 (-48.5, 56.825) -> (-45, 56.825) projected
  line L136 (-86.825, 60) -> (-75, 60) projected
  line L137 (-86.825, 55) -> (-86.825, 60) projected
  line L138 (-86.825, -60) -> (-86.825, -55) projected
  line L139 (-86.825, -60) -> (-75, -60) projected
  line L140 (75, -60) -> (86.825, -60) projected
  line L141 (86.825, -55) -> (86.825, -60) projected
  line L142 (86.825, 60) -> (86.825, 55) projected
  line L143 (75, 60) -> (86.825, 60) projected
  point P0 (0, 0)
  dimension "d136" = 1.905
  dimension "d137" = 1.905
  dimension "d138" = 11.43
  dimension "d139" = 3.81
  constraints: 8 end point, 2 parallel, 1 horizontal, 1 perpendicular
  measures "d136" distance from line of A0.centre L3
  measures "d137" distance from line of A0.centre L0
  measures "d138" distance of L0.start L0.end
  measures "d139" distance of L0.end L1.end
extrude "Extrusion7" cut sketch "Sketch15" against normal through all contours L3 L2 L1 L0
equation "\"d1\" = height - 2 * materialThickness"
equation "\"d2\" = materialThickness"
equation "\"d84\" = notchWidth"
equation "\"d86\" = materialThickness"
equation "\"d91\" = 2 * notchWidth"
equation "\"d92\" = materialThickness"
equation "\"d94\" = notchWidth"
equation "\"d100\" = 0.5 * notchWidth"
equation "\"d99\" = 2 * notchWidth"
equation "\"d4\" = axleHeight"
equation "\"d12\" = 0.5 * spoolDiameter - materialThickness"
equation "\"d5\" = bearingOd"
equation "\"d41\" = nutTrapwidth"
equation "\"d42\" = nutTrapDepth"
equation "\"d77\" = magnetDiameter"
equation "\"materialThickness\" = 3.175"
equation "\"laserKerf\" = 0.1"
equation "\"cardPinDiameter\" = 3"
equation "\"cardHeight\" = 53.98"
equation "\"cardSelected\" = 1"
equation "\"cardFillet\" = 2.88"
equation "\"centeralShaftDiameter\" = 8"
equation "\"cardThickness\" = 0.76"
equation "\"cardWidth\" = 85.6"
equation "\"cardClearence\" = 0.5"
equation "\"bearingWidth\" = 8"
equation "\"bearingOd\" = 22"
equation "\"axleHeight\" = 95"
equation "\"nutTrapDepth\" = 2.5"
equation "\"nutTrapClearence\" = 2"
equation "\"nutTrapwidth\" = 5.5"
equation "\"magnetLength\" = 3"
equation "\"magnetDiameter\" = 6"
equation "\"magnetProtusion\" = 0.25"
equation "\"notchWidth\" = 10"
equation "\"spoolThickness\" = 5.588"
equation "\"height\" = 180"
equation "\"spoolDiameter\" = 90"
body "Solid1"
